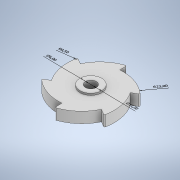
# Autodesk Inventor part: Część12
Saved by Autodesk Inventor 2021 (Build 250183000, 183)
## iProperties
Created: 2023-10-06
Part Number: Część12
Material: Ogólny
Document SubType Name: Modeling
Designer: Jakub
Density: 1 g/cm^3
Appearance: Domyślna
Author: Jakub
Autodesk Inventor part; units mm, degrees
ref_plane "YZ Plane" through (0, 0, 0) normal (1, 0, 0) x (0, 1, 0)
ref_plane "XZ Plane" through (0, 0, 0) normal (0, 1, 0) x (-1, 0, 0)
ref_plane "XY Plane" through (0, 0, 0) normal (0, 0, 1) x (1, 0, 0)
sketch "Szkic1" plane through (0, 0, 0) normal (0, 1, 0) x (-1, 0, 0)
  circle A0 centre (0, 0) radius 20
  circle A1 centre (0, 0) radius 16
  line L0 (0, 0) -> (-17.3205, -10)
  line L1 (0, 0) -> (20, 0) construction
  line L2 (0, 0) -> (-17.3205, 10)
  line L3 (0, 0) -> (20, 0) construction
  line L4 (0, 0) -> (0, 20)
  line L5 (0, 0) -> (20, 0) construction
  line L6 (0, 0) -> (17.3205, 10)
  line L7 (0, 0) -> (17.3205, -10)
  line L8 (0, 0) -> (0, -20)
  line L9 (0, -20) -> (13.8564, -8)
  line L10 (17.3205, -10) -> (13.8564, 8)
  line L11 (17.3205, 10) -> (0, 16)
  line L12 (0, 20) -> (-13.8564, 8)
  line L13 (-17.3205, 10) -> (-13.8564, -8)
  line L14 (-17.3205, -10) -> (0, -16)
  line L15 (0, -20) -> (0, -16)
  line L16 (17.3205, -10) -> (13.8564, -8)
  line L17 (17.3205, 10) -> (13.8564, 8)
  line L18 (0, 16) -> (0, 20)
  arc A2 (-17.3205, -10) -> (0, -16) centre (-1.7553, 6.9329) ccw
  arc A3 (0, -20) -> (13.8564, -8) centre (-6.8817, 1.9463) ccw
  arc A4 (17.3205, -10) -> (13.8564, 8) centre (-5.1264, -4.9866) ccw
  arc A5 (17.3205, 10) -> (0, 16) centre (1.7553, -6.9329) ccw
  arc A6 (-17.3205, 10) -> (-13.8564, -8) centre (5.1264, 4.9866) ccw
  arc A7 (0, 20) -> (-13.8564, 8) centre (6.8817, -1.9463) ccw
  dimension "d0" = 40
  dimension "d1" = 32
  dimension "d2" = 150
  dimension "d3" = 150
  dimension "d4" = 90
  dimension "d5" = 23
  dimension "d6" = 23
  dimension "d7" = 23
  dimension "d8" = 23
  dimension "d9" = 23
  dimension "d10" = 23
  constraints: 38 end point, 24 point on circle, 8 centre point, 6 point on line, 4 collinear, 3 equal length, 3 horizontal, 2 coincident, 1 perpendicular
  measures "d0" diameter of A0
  measures "d1" diameter of A1
  measures "d2" angle of L0 L1
  measures "d3" angle of L3 L2
  measures "d4" angle of L5 L4
  measures "d5" radius of A2
  measures "d6" radius of A3
  measures "d7" radius of A4
  measures "d8" radius of A5
  measures "d9" radius of A6
  measures "d10" radius of A7
extrude "Wyciągnięcie proste1" add sketch "Szkic1" along normal blind 6 contours L6 A1 L11 | L11 A1 A5 | L7 A1 L10 | L10 A1 A4 | L4 A1 L12 | L12 A1 A7 | L6 L4 L11 A1 | L10 A1 L7 L6 | A1 L10 | L11 A1 | L4 L2 L12 A1 | L8 A1 L9 | L9 A1 A3 | L9 A1 L8 L7 | A1 L9 | L2 A1 L13 | L13 A1 A6 | L12 A1 | L2 L0 L13 A1 | L8 L14 A1 L0 | L0 A1 L14 | L14 A1 A2 | A1 L14 | L13 A1
fillet "Zaokrąglenie1" radius 0.5 6 edges at (0, 3, -20) (17.3205, 3, -10) (17.3205, 3, 10) (0, 3, 20) (-17.3205, 3, 10) (-17.3205, 3, -10)
sketch "Szkic2" plane through (0, 6, 0) normal (0, 1, 0) x (1, 0, 0)
  circle A0 centre (0, 0) radius 6
  dimension "d14" = 12
  constraints: 1 centre point, 1 coincident
  measures "d14" diameter of A0
extrude "Wyciągnięcie proste2" add sketch "Szkic2" along normal blind 1
sketch "Szkic3" plane through (0, 0, 0) normal (0, -1, 0) x (1, 0, 0)
  circle A0 centre (0, 0) radius 6
  dimension "d17" = 12
  constraints: 1 centre point, 1 coincident
  measures "d17" diameter of A0
extrude "Wyciągnięcie proste3" cut sketch "Szkic3" against normal blind 1
sketch "Szkic4" plane through (0, 7, 0) normal (0, 1, 0) x (1, 0, 0)
  circle A0 centre (0, 0) radius 3
  dimension "d20" = 6
  constraints: 1 centre point, 1 coincident
  measures "d20" diameter of A0
extrude "Wyciągnięcie proste4" cut sketch "Szkic4" against normal blind 6
